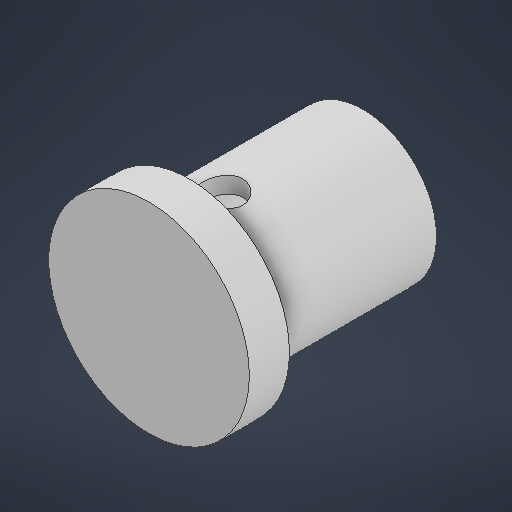
# Autodesk Inventor part: SAFRS-P-0060
Saved by Autodesk Inventor 2026.2 (Build 302298000, 298)
## iProperties
Created: 2025-12-01
Part Number: SAFRS-P-0060
Material: 일반
Document SubType Name: Modeling
Designer: jaewook
Density: 1 g/cm^3
Appearance: 기본값
Author: jaewook
Title: Stopper
Autodesk Inventor part; units mm, degrees
ref_plane "YZ Plane" through (0, 0, 0) normal (1, 0, 0) x (0, 1, 0)
ref_plane "XZ Plane" through (0, 0, 0) normal (0, 1, 0) x (-1, 0, 0)
ref_plane "XY Plane" through (0, 0, 0) normal (0, 0, 1) x (1, 0, 0)
sketch "스케치1" plane through (0, 0, 0) normal (0, 0, 1) x (1, 0, 0)
  circle A0 centre (0, 0) radius 5.5
  circle A1 centre (0, 0) radius 4.3
  dimension "d0" = 11
  dimension "d1" = 8.6
  constraints: 2 centre point, 2 coincident
  measures "d0" diameter of A0
  measures "d1" diameter of A1
extrude "돌출1" add sketch "스케치1" along normal blind 13
sketch "스케치2" plane through (0, 0, 13) normal (0, 0, 1) x (1, 0, 0)
  circle A0 centre (0, 0) radius 4.3 projected
  circle A1 centre (0, 0) radius 7.5
  dimension "d4" = 15
  constraints: 1 centre point, 1 coincident
  measures "d4" diameter of A1
extrude "돌출2" add sketch "스케치2" along normal blind 3 contours A0 | A1
sketch "스케치3" plane through (0, 0, 0) normal (1, 0, 0) x (0, 1, 0)
  line L0 (7.4799, 10.5) -> (-8.5589, 10.5)
  line L1 (-8.5589, 10.5) -> (-8.5589, 12)
  line L2 (-8.5589, 12) -> (7.4799, 12)
  line L3 (7.4799, 12) -> (7.4799, 10.5)
  line L4 (7.5, 13) -> (-7.5, 13) projected
  point P0 (0, 0)
  dimension "d7" = 1.5
  dimension "d10" = 2.5
  constraints: 8 end point, 2 parallel, 1 horizontal, 1 perpendicular
  measures "d7" distance between parallel lines of L2 L0
  measures "d10" distance from line of L0.start L4
revolve "회전1" cut sketch "스케치3" angle 360 about axis through (0, 7.4799, 10.5) along (0, -1, 0)
